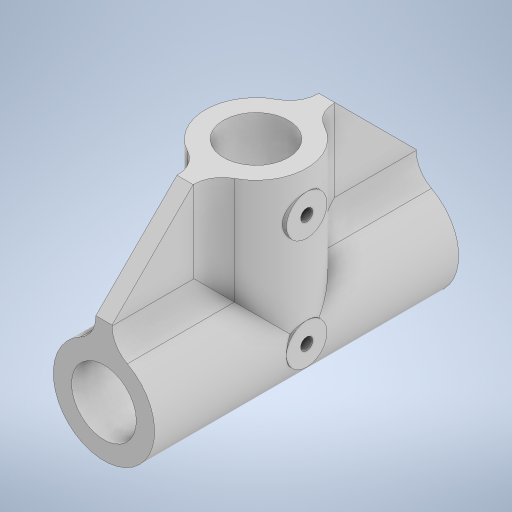
# Autodesk Inventor part: LegTeeJoint2.5
Saved by Autodesk Inventor 2023 (Build 270158000, 158)
## iProperties
Created: 2022-12-09
Part Number: LegTeeJoint2.5
Material: Generic
Document SubType Name: Modeling
Designer: Administrator
Density: 1 g/cm^3
Appearance: Default
Author: Administrator
Autodesk Inventor part; units mm, degrees
ref_plane "YZ Plane" through (0, 0, 0) normal (1, 0, 0) x (0, 1, 0)
ref_plane "XZ Plane" through (0, 0, 0) normal (0, 1, 0) x (-1, 0, 0)
sketch "Sketch1" plane through (0, 0, 0) normal (0, 0, 1) x (1, 0, 0)
  arc A0 (0, 12.5) -> (-2, 12.339) centre (0, 0) ccw construction
  line L0 (0, 12.5) -> (0, 37.5) construction
  line L1 (0, 37.5) -> (-2, 37.5)
  line L2 (-2, 37.5) -> (-2, 12.339)
  line L3 (0, 37.5) -> (2, 37.5)
  line L4 (2, 37.5) -> (2, 12.339)
  arc A1 (2, 12.339) -> (0, 12.5) centre (0, 0) ccw construction
  arc A2 (-2, 12.339) -> (2, 12.339) centre (0, 0) ccw
  dimension "d1" = 25
  dimension "d14" = 25
  dimension "d15" = 2
  dimension "d16" = 2
  constraints: 10 end point, 6 point on circle, 3 centre point, 2 perpendicular, 1 horizontal, 1 point on line, 1 vertical
  measures "d1" diameter of A0
  measures "d14" distance of L0.start L0.end
  measures "d15" distance of L0.end L1.end
  measures "d16" distance of L0.end L3.end
extrude "Extrusion1" add sketch "Sketch1" along normal blind 75
sketch "Sketch5" plane through (-2, 37.5, 0) normal (0, 1, 0) x (1, 0, 0)
  line L0 (4, 0) -> (0, 0) construction
  line L1 (4, -75) -> (0, -75) construction
  line L2 (0, 0) -> (4, -75) construction
  circle A0 centre (2, -37.5) radius 12.5
  point P0 (2, 0)
  constraints: 2 end point, 1 centre point
extrude "Extrusion4" add sketch "Sketch5" against normal up to surface
chamfer "Chamfer1" distance 20 angle 45 2 edges at (0, 37.5, 75) (0, 37.5, 0)
fillet "Fillet1" radius 7 8 edges at (2, 24.9195, 25.161) (2, 24.9195, 49.839) (2, 12.339, 62.4195) (-2, 24.9195, 25.161) (-2, 24.9195, 49.839) (-2, 12.339, 62.4195) (-2, 12.339, 12.5805) (2, 12.339, 12.5805)
ref_plane "Work Plane2" through (12.5, 37.5, 37.5) normal (1, 0, 0) x (0, 0, -1)
sketch "Sketch8" plane through (12.5, 37.5, 37.5) normal (1, 0, 0) x (0, 0, -1)
  line L0 (11.089, 0) -> (-11.089, 0) construction
  line L1 (0, 0) -> (0, -10) construction
  circle A0 centre (0, -10) radius 5
  line L2 (0, -37.5) -> (11.089, -26.411) projected
  circle A1 centre (0, -37.5) radius 5
  point P0 (37.5, -37.5)
  dimension "d31" = 10
  dimension "d32" = 10
  dimension "d33" = 10
  constraints: 2 centre point, 2 end point, 1 coincident, 1 midpoint, 1 vertical
  measures "d31" distance of L1.start L1.end
  measures "d32" diameter of A0
  measures "d33" diameter of A1
extrude "Extrusion6" add sketch "Sketch8" against normal blind 25
sketch "Sketch6" plane through (-2, 37.5, 0) normal (0, 1, 0) x (1, 0, 0)
  circle A0 centre (2, -37.5) radius 8
  point P0 (2, 0)
  dimension "d20" = 16
  constraints: 1 centre point
  measures "d20" diameter of A0
extrude "Extrusion5" cut sketch "Sketch6" against normal blind 25
sketch "Sketch4" plane through (0, 0, 75) normal (0, 0, 1) x (1, 0, 0)
  circle A0 centre (0, 0) radius 8
  arc A1 (-5.7692, 11.089) -> (5.7692, 11.089) centre (0, 0) ccw projected
  dimension "d30" = 16
  constraints: 1 centre point, 1 coincident, 1 concentric
  measures "d30" diameter of A0
extrude "Extrusion3" cut sketch "Sketch4" against normal up to next
sketch "Sketch9" plane through (12.5, 37.5, 37.5) normal (1, 0, 0) x (0, 0, -1)
  arc A0 (0, -5) -> (0, -15) centre (0, -10) ccw projected
  circle A1 centre (0, -10) radius 1.5
  circle A2 centre (0, -37.5) radius 1.5
  point P0 (37.5, -37.5)
  dimension "d36" = 3
  dimension "d37" = 3
  constraints: 2 centre point, 1 coincident
  measures "d36" diameter of A1
  measures "d37" diameter of A2
extrude "Extrusion7" cut sketch "Sketch9" against normal up to surface (25 mm away)
body "Solid1"
